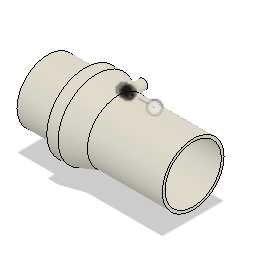
Oxygen Mixer V1 (Autodesk Fusion 360 design; units mm, degrees)
Autodesk Fusion 360 part; units mm, degrees
note: some values were not read from the file. Set by a fixed rule: which sketch regions a step uses.
sketch "Sketch7" plane through (0, 0, 0) normal (0, 1, 0) x (1, 0, 0)
  line L0 (-5.6796, 17.9856) -> (28.2056, 6.3689)
  line L1 (28.2056, 6.3689) -> (27.7191, 4.95)
  line L2 (27.7191, 4.95) -> (-1.5962, 15)
  line L3 (-1.5962, 15) -> (-26.6796, 15)
  line L4 (-26.6796, 15) -> (-26.6796, 16.5)
  line L5 (-5.6796, 17.9856) -> (-5.6796, 19.5)
  line L6 (-5.6796, 19.5) -> (-0.8463, 19.5)
  line L7 (-0.8463, 19.5) -> (31.2048, 8.5121)
  line L8 (31.2048, 8.5121) -> (31.2056, 4.95)
  line L9 (31.2056, 4.95) -> (32.2056, 4.9502)
  line L10 (32.2056, 4.9502) -> (32.2047, 9.2265)
  line L11 (-0.6796, 20.5) -> (-6.6796, 20.5)
  line L12 (-6.6796, 20.5) -> (-6.6796, 16.5)
  line L13 (10.9882, 16.5) -> (50.9882, 16.5)
  line L14 (50.9882, 16.5) -> (50.9882, 15)
  line L15 (50.9882, 15) -> (15.3636, 15)
  line L16 (-22.2609, 0) -> (38.4517, 0) construction
  line L17 (-26.6796, 16.5) -> (-6.6796, 16.5)
  line L18 (32.2047, 9.2265) -> (15.3636, 15)
  line L19 (10.9882, 16.5) -> (-0.6796, 20.5)
  line L20 (27.7191, 4.95) -> (31.2056, 4.95) construction
  dimension "d24" = 15
  dimension "d25" = 1.5
  dimension "d26" = 1
  dimension "d27" = 1
  dimension "d28" = 1
  dimension "d29" = 1
  dimension "d30" = 3
  dimension "d31" = 20
  dimension "d32" = 40
  dimension "d33" = 4.95
  dimension "d34" = 3
  dimension "d42" = 6
  constraint horizontal L17
  constraint perpendicular L0 L1
  constraint perpendicular L1 L2
  constraint parallel L3 L17
  constraint perpendicular L5 L17
  constraint perpendicular L8 L9
  constraint perpendicular L9 L10
  constraint horizontal L11
  constraint perpendicular L12 L17
  constraint coincident L13.start L18
  constraint parallel L3 L13
  constraint perpendicular L13 L14
  constraint perpendicular L14 L15
  constraint horizontal L16
  constraint coincident L16 origin
  constraint collinear L18 L19
  constraint coincident L11.end L12.start
  constraint coincident L5.end L6.start
  constraint horizontal L6
  constraint vertical L4
  constraint equal L4 L14
  constraint parallel L7 L18
  constraint equal L1 L14
  constraint horizontal L20
  constraint coincident L8.end L9.start
  constraint parallel L0 L7
  constraint collinear L3 L15
  measures "d24" distance of L15 L16
  measures "d25" distance of L13.end L14.end
  measures "d26" distance of L8.end L9.end
  measures "d27" distance of L7 L19
  measures "d28" distance of L6 L11
  measures "d29" distance of L5 L12
  measures "d30" distance of L0.end L7
  measures "d31" distance of L4.end L12.end
  measures "d32" distance of L13.start L13.end
  measures "d33" distance of L1.end L16
  measures "d34" horizontal distance of L0.end L8.end
  measures "d42" distance of L11.start L11.end
revolve "Revolve1" add sketch "Sketch7" angle 360 about axis through (-22.2609, 0, 0) along (1, 0, 0) makes body 1 in component "Mixer"
ref_plane "WorkPlane5" through (-3.5133, 0, -20.5) normal (0, 0, -1) x (0, -1, 0)
sketch "Sketch9" plane through (-5.5333, 0, -20.5) normal (0, 0, -1) x (1, 0, 0)
  circle A0 centre (1.3536, 0) radius 1.5
  circle A1 centre (1.3536, 0) radius 2.5
  line L0 (0, 0) -> (15.4346, 0) construction
  point P0 (-1.1464, 0)
  point P1 (-1.1464, 0)
  dimension "d36" = 3
  dimension "d37" = 1
  constraint concentric A0 A1
  constraint coincident L0.start origin
  constraint horizontal L0
  constraint coincident A0.centre L0
  constraint coincident L0 P1
  constraint coincident A1 P1
  constraint coincident P1 P0
  measures "d36" diameter of A0
  measures "d37" distance of A0 A1
extrude "Extrude2" cut sketch "Sketch9" along normal up to surface contours A0 end surface at (-4.0685, -0.972, -19.4758) on bodies 1 bodies 1 in component "Mixer"
extrude "Extrude2'" add sketch "Sketch9" along normal blind 8 separate body makes body 2
copy_body "CutPasteBodies2" bodies 2 removing the originals makes body 3 in component "Mixer"
component "Mixer" placed x (1, 0, 0) y (0, 1, 0) z (0, 0, 1) at (0, 0, 0)
